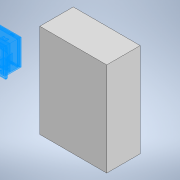
# Autodesk Inventor part: casing
Saved by Autodesk Inventor 2022.1 (Build 261234020, 234B)
## iProperties
Created: 2022-01-26
Part Number: casing
Material: Generic
Document SubType Name: Modeling
Designer: logic
Density: 1 g/cm^3
Appearance: Default
Author: logic
Autodesk Inventor part; units mm, degrees
ref_plane "YZ Plane" through (0, 0, 0) normal (1, 0, 0) x (0, 1, 0)
ref_plane "XZ Plane" through (0, 0, 0) normal (0, 1, 0) x (-1, 0, 0)
ref_plane "XY Plane" through (0, 0, 0) normal (0, 0, 1) x (1, 0, 0)
sketch "Sketch1" plane through (0, 0, 0) normal (0, 0, 1) x (1, 0, 0)
  line L0 (-50, 60) -> (50, 60)
  line L1 (50, 60) -> (50, -60)
  line L2 (50, -60) -> (-50, -60)
  line L3 (-50, -60) -> (-50, 60)
  point P0 (0, 0)
  dimension "d0" = 100
  dimension "d1" = 120
  dimension "d2" = 60
  dimension "d3" = 50
  constraints: 8 end point, 2 parallel, 1 horizontal, 1 perpendicular
  measures "d0" distance between parallel lines of L1 L3
  measures "d1" distance between parallel lines of L0 L2
  measures "d2" distance from line of L2 point (0, 0)
  measures "d3" distance from line of point (0, 0) L3
extrude "Extrusion1" add sketch "Sketch1" along normal mid plane 50
sketch "Sketch2" plane through (0, 0, -25) normal (0, 0, -1) x (-1, 0, 0)
  line L0 (-45, 55) -> (45, 55)
  line L1 (45, 55) -> (45, -60)
  line L2 (45, -60) -> (-45, -60)
  line L3 (-45, -60) -> (-45, 55)
  line L4 (-50, -60) -> (-50, 60) projected
  line L5 (-50, 60) -> (50, 60) projected
  line L6 (-50, 60) -> (50, 60)
  line L7 (50, -60) -> (-50, -60) projected
  line L8 (50, 60) -> (50, -60)
  line L9 (50, -60) -> (-50, -60)
  line L10 (-50, -60) -> (-50, 60)
  point P0 (0, 0)
  point P1 (0, -60)
  dimension "d6" = 5
  dimension "d7" = 5
  dimension "d8" = 5
  constraints: 16 end point, 3 equal length, 3 perpendicular, 2 horizontal, 2 midpoint
  measures "d6" distance between parallel lines of L0 L5
  measures "d7" distance between parallel lines of L3 L4
  measures "d8" distance between parallel lines of L8 L1
extrude "Extrusion2" cut sketch "Sketch2" against normal blind 45 contours L0 L1 L2 L3
body "Solid1"
